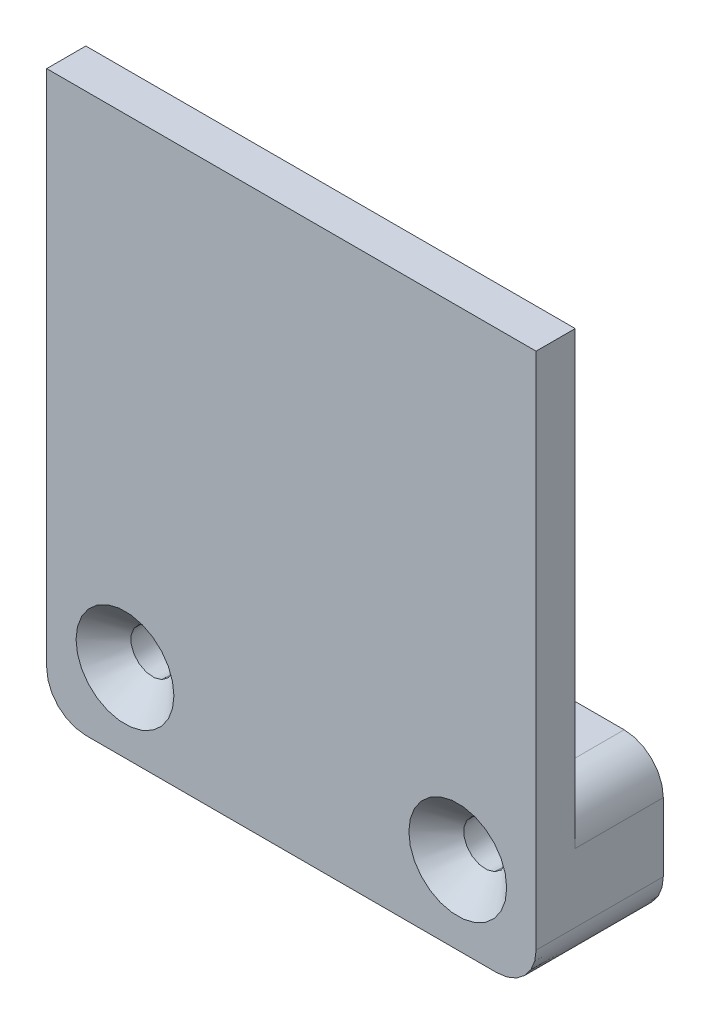
# Autodesk Inventor part: Sliderhalter
Saved by Autodesk Inventor 2025 (Build 290162010, 162A)
## iProperties
Created: 2024-11-26
Part Number: Sliderhalter
Material: PC/ABS-Kunststoff, 3DDruck, PLA
Document SubType Name: Modeling
Designer: Admin
Density: 1.1 g/cm^3
Appearance: Glatt - Weiß(2)
Author: Admin
Autodesk Inventor part; units mm, degrees
ref_plane "YZ Plane" through (0, 0, 0) normal (1, 0, 0) x (0, 1, 0)
ref_plane "XZ Plane" through (0, 0, 0) normal (0, 1, 0) x (-1, 0, 0)
ref_plane "XY Plane" through (0, 0, 0) normal (0, 0, 1) x (1, 0, 0)
sketch "Skizze1" plane through (0, 0, 0) normal (0, 0, 1) x (1, 0, 0)
  line L0 (75.1333, -4.3546) -> (75.1333, -11.8546)
  line L1 (75.1333, -11.8546) -> (50.1333, -11.8546)
  line L2 (50.1333, -11.8546) -> (50.1333, -4.3546)
  line L3 (50.1333, -4.3546) -> (75.1333, -4.3546)
  point P0 (0, 0)
  dimension "d1" = 7.5
  dimension "d2" = 25
  constraints: 8 end point, 2 perpendicular, 1 horizontal, 1 parallel
  measures "d1" distance of L0.end L0.start
  measures "d2" distance of L0.start L2.end
extrude "Extrusion1" add sketch "Skizze1" along normal blind 4.5
sketch "Skizze2" plane through (0, 0, 4.5) normal (0, 0, 1) x (1, 0, 0)
  line L0 (75.1333, 16.6454) -> (50.1333, 16.6454)
  line L1 (50.1333, 16.6454) -> (50.1333, -4.3546)
  line L2 (75.1333, -4.3546) -> (75.1333, 16.6454)
  line L3 (50.1333, -11.8546) -> (75.1333, -11.8546) projected
  line L4 (75.1333, -11.8546) -> (75.1333, -4.3546) projected
  line L5 (50.1333, -4.3546) -> (50.1333, -11.8546) projected
  point P0 (0, 0)
  dimension "d25" = 28.5
  constraints: 6 end point, 1 collinear, 1 perpendicular, 1 vertical
  measures "d25" distance between parallel lines of L0 L3
extrude "Extrusion2" add sketch "Skizze2" along normal blind 2
sketch "Skizze3" plane through (0, 0, 6.5) normal (0, 0, 1) x (1, 0, 0)
  line L0 (50.1333, 16.6454) -> (50.1333, -11.8546) projected
  line L1 (54.1333, -7.8546) -> (50.1333, -7.8546) construction
  line L2 (54.1333, -7.8546) -> (54.1333, -11.8546) construction
  line L3 (71.1333, -7.8546) -> (71.1333, -11.8546) construction
  line L4 (71.1333, -7.8546) -> (75.1333, -7.8546) construction
  line L5 (50.1333, -11.8546) -> (75.1333, -11.8546) construction
  line L6 (75.1333, -11.8546) -> (75.1333, 16.6454) construction
  point P0 (0, 0)
  dimension "d26" = 4
  constraints: 8 end point, 4 point on line, 3 equal length, 2 vertical, 1 horizontal, 1 perpendicular
  measures "d26" distance from line of L0 L1.start
hole "Bohrung1" at (54.1333, -7.8546, 6.5) at (71.1333, -7.8546, 6.5) direction (0, 0, -1) diameter 2.2 end through all countersink diameter 5 countersink angle 90
fillet "Rundung1" radius 2 4 edges at (50.1333, -11.8546, 3.25) (75.1333, -11.8546, 3.25) (75.1333, -4.3546, 2.25) (50.1333, -4.3546, 2.25)
